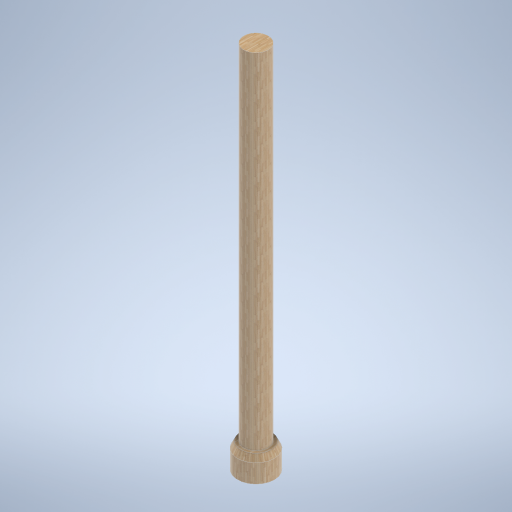
# Autodesk Inventor part: Tower
Saved by Autodesk Inventor 2023 (Build 270158000, 158)
## iProperties
Created: 2023-10-27
Part Number: Tower
Material: Wood (Maple)
Document SubType Name: Modeling
Designer: Admin
Density: 0.67 g/cm^3
Appearance: Natural Maple - Glossy Dark Tint
Author: Admin
Autodesk Inventor part; units mm, degrees
ref_plane "YZ Plane" through (0, 0, 0) normal (1, 0, 0) x (0, 1, 0)
ref_plane "XZ Plane" through (0, 0, 0) normal (0, 1, 0) x (-1, 0, 0)
ref_plane "XY Plane" through (0, 0, 0) normal (0, 0, 1) x (1, 0, 0)
sketch "Sketch1" plane through (0, 0, 0) normal (0, 0, 1) x (1, 0, 0)
  line L0 (0, 0) -> (750, 0)
  line L1 (750, 0) -> (750, 750)
  line L2 (750, 750) -> (625, 1000)
  line L3 (625, 1000) -> (500, 1000)
  line L4 (500, 1000) -> (500, 15000)
  line L5 (500, 15000) -> (0, 15000)
  line L6 (0, 15000) -> (0, 0)
  dimension "d0" = 750
  dimension "d1" = 750
  dimension "d2" = 15000
  dimension "d3" = 250
  dimension "d4" = 125
  dimension "d5" = 500
  constraints: 14 end point, 4 perpendicular, 1 horizontal, 1 parallel
  measures "d0" distance of L0.start L0.end
  measures "d1" distance of L0.end L1.end
  measures "d2" distance of L5.end L0.start
  measures "d3" vertical distance of L2.end L1.end
  measures "d4" distance of L3.end L2.end
  measures "d5" distance of L4.end L5.end
revolve "Revolution1" add sketch "Sketch1" angle 360 about axis through (0, 15000, 0) along (0, -1, 0)
body "Solid1"
